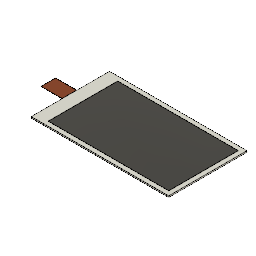
METEOSTANICE VNITRNI SESTAVA v6 (Autodesk Fusion 360 archive; units mm, degrees)
design "E-ink displej"
Autodesk Fusion 360 part; units mm, degrees
(part 1 of 2)
sketch "Sketch1" plane through (0, 0, 0) normal (0, 0, 1) x (1, 0, 0)
  line L0 (0, 0) -> (92.99, 0)
  line L1 (92.99, 0) -> (92.99, 53)
  line L2 (92.99, 53) -> (0, 53)
  line L3 (0, 53) -> (0, 0)
  dimension "d1" = 92.99
  dimension "d2" = 53
  constraint horizontal L0
  constraint vertical L1
  constraint horizontal L2
  constraint vertical L3
  constraint coincident L0.start L3.end
  measures "d1" distance of L0.start L0.end
  measures "d2" distance of L0.start L2.end
extrude "Extrude1" add sketch "Sketch1" along normal blind 1 makes body 1
sketch "Sketch2" plane through (0, 0, 1) normal (0, 0, 1) x (-1, 0, 0)
  line L0 (0, -53) -> (0, 0)
  line L1 (0, 0) -> (-92.99, 0)
  line L2 (-92.99, 0) -> (-92.99, -53)
  line L3 (-92.99, -53) -> (0, -53)
  line L4 (-8.5, -3) -> (-90.04, -3)
  line L5 (-90.04, -3) -> (-90.04, -50.04)
  line L6 (-90.04, -50.04) -> (-8.5, -50.04)
  line L7 (-8.5, -50.04) -> (-8.5, -3)
  dimension "d5" = 81.54
  dimension "d6" = 47.04
  dimension "d7" = 8.5
  dimension "d8" = 3
  constraint horizontal L4
  constraint vertical L5
  constraint horizontal L6
  constraint vertical L7
  measures "d5" distance of L4.start L4.end
  measures "d6" distance of L4.start L6.end
  measures "d7" horizontal distance of L0.end L4.start
  measures "d8" vertical distance of L0.end L4.start
extrude "Extrude2" add sketch "Sketch2" along normal blind 0.001 separate body contours L4 L5 L6 L7 makes body 2
sketch "Sketch3" plane through (0, 0, 0) normal (-1, 0, 0) x (0, -1, 0)
  line L0 (-53, 0) -> (0, 0)
  line L1 (0, 0) -> (0, 1)
  line L2 (0, 1) -> (-53, 1)
  line L3 (-53, 1) -> (-53, 0)
  line L4 (-26.5, 1) -> (-26.5, 0)
  line L5 (-26.5, 0.3186) -> (-21.5, 0.3186)
  line L6 (-21.5, 0.3186) -> (-31.5, 0.3186)
  line L7 (-31.5, 0.3186) -> (-31.5, 0.4186)
  line L8 (-31.5, 0.4186) -> (-21.5, 0.4186)
  line L9 (-21.5, 0.4186) -> (-21.5, 0.3186)
  dimension "d11" = 5
  dimension "d12" = 10
  dimension "d13" = 0.1
  constraint midpoint L2 L4.start
  constraint midpoint L0 L4.end
  constraint coincident L4 L5.start
  constraint perpendicular L4 L5
  constraint horizontal L6
  constraint vertical L7
  constraint horizontal L8
  constraint vertical L9
  measures "d11" distance of L5.start L5.end
  measures "d12" distance of L5.end L6.end
  measures "d13" distance of L5.end L8.end
extrude "Extrude3" add sketch "Sketch3" along normal blind 15 separate body contours L4 L6 L7 L8 | L4 L5 L6 L8 L9 makes body 3

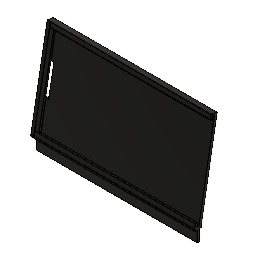
design "meteostanice_vnitrni-uchytDisplej"
Autodesk Fusion 360 part; units mm, degrees
sketch "Sketch1" plane through (0, 0, 0) normal (1, 0, 0) x (0, 1, 0)
  line L0 (0, 0) -> (1.5, 0)
  line L1 (0, 0) -> (0, 6.8)
  line L2 (1.5, 0) -> (1.5, 6.8)
  line L3 (0, 6.8) -> (-1.5, 6.8)
  line L4 (-1.5, 6.8) -> (-1.5, 7.8)
  line L5 (1.5, 6.8) -> (2.5, 6.8)
  line L6 (2.5, 6.8) -> (2.5, 7.8)
  line L7 (2.5, 7.8) -> (-1.5, 7.8)
  line L8 (-1.5, 7.8) -> (-1.0311, 10.459)
  line L9 (-1.0311, 10.459) -> (-0.0463, 10.2853)
  line L10 (2.5, 7.8) -> (11.9465, 61.3735)
  line L11 (2.5, 7.8) -> (56, 7.8) construction
  line L12 (2.5, 7.8) -> (1.0228, 8.0605)
  line L13 (2.5, 7.8) -> (3.5, 7.8) construction
  line L14 (1.0228, 8.0605) -> (10.4692, 61.634)
  line L15 (1.0228, 8.0605) -> (55.0152, 8.0605) construction
  line L16 (11.9465, 61.3735) -> (10.4692, 61.634)
  line L17 (1.0228, 8.0605) -> (-0.159, 8.2689)
  line L18 (-0.159, 8.2689) -> (0.1893, 10.2438)
  line L19 (0.1893, 10.2438) -> (-0.0463, 10.2853)
  line L20 (10.4692, 61.634) -> (9.2875, 61.8424)
  line L21 (9.2875, 61.8424) -> (8.8186, 59.1834)
  line L22 (10.4692, 61.634) -> (10.2956, 60.6492)
  line L23 (10.2956, 60.6492) -> (9.1138, 60.8576)
  line L24 (8.8186, 59.1834) -> (7.8338, 59.3571)
  line L25 (9.2875, 61.8424) -> (8.3027, 62.016)
  line L26 (8.3027, 62.016) -> (7.8338, 59.3571)
  dimension "d1" = 1.5
  dimension "d2" = 6.8
  dimension "d3" = 6.8
  dimension "d4" = 1.5
  dimension "d5" = 1
  dimension "d6" = 1
  dimension "d7" = 1
  dimension "d8" = 2.7
  dimension "d9" = 80
  dimension "d10" = 1
  dimension "d11" = 80
  dimension "d12" = 54.4
  dimension "d13" = 170
  dimension "d14" = 1.5
  dimension "d15" = 80
  dimension "d16" = 54.4
  dimension "d17" = 1.2
  dimension "d18" = 1.2
  dimension "d19" = 2.7
  dimension "d20" = 1
  dimension "d21" = 1
  dimension "d22" = 1
  constraint coincident L0.start L1.start
  constraint horizontal L0
  constraint perpendicular L0 L1
  constraint perpendicular L0 L2
  constraint perpendicular L1 L3
  constraint perpendicular L3 L4
  constraint perpendicular L2 L5
  constraint perpendicular L5 L6
  constraint perpendicular L8 L9
  constraint horizontal L11
  constraint horizontal L13
  constraint horizontal L15
  constraint perpendicular L14 L17
  constraint perpendicular L17 L18
  constraint perpendicular L18 L19
  constraint perpendicular L14 L20
  constraint perpendicular L20 L21
  constraint perpendicular L16 L22
  constraint coincident L21 L23.end
  constraint perpendicular L21 L23
  constraint perpendicular L21 L24
  constraint perpendicular L21 L25
  measures "d1" distance of L0.start L0.end
  measures "d2" distance of L0.start L1.end
  measures "d3" distance of L0.end L2.end
  measures "d4" distance of L1.end L3.end
  measures "d5" distance of L3.end L4.end
  measures "d6" distance of L2.end L5.end
  measures "d7" distance of L5.end L6.end
  measures "d8" distance of L4.end L8.end
  measures "d9" angle of L7 L8
  measures "d10" distance of L8.end L9.end
  measures "d11" angle of L10 L11
  measures "d12" distance of L6.end L10.end
  measures "d13" angle of L12 L13
  measures "d14" distance of L6.end L12.end
  measures "d15" angle of L14 L15
  measures "d16" distance of L12.end L14.end
  measures "d17" distance of L12.end L17.end
  measures "d18" distance of L14.end L20.end
  measures "d19" distance of L20.end L21.end
  measures "d20" distance of L14.end L22.end
  measures "d21" distance of L21.end L24.end
  measures "d22" distance of L20.end L25.end
extrude "Extrude1" add sketch "Sketch1" along normal blind 95.5
sketch "Sketch2" plane through (0, 0, 0) normal (-1, 0, 0) x (0, -1, 0)
  line L0 (-1.5, 0) -> (0, 0)
  line L1 (0, 0) -> (0, 6.8)
  line L2 (0, 6.8) -> (1.5, 6.8)
  line L3 (1.5, 6.8) -> (1.5, 7.8)
  line L4 (1.5, 7.8) -> (1.0311, 10.459)
  line L5 (1.0311, 10.459) -> (-0.1893, 10.2438)
  line L6 (-0.1893, 10.2438) -> (0.159, 8.2689)
  line L7 (0.159, 8.2689) -> (-1.0228, 8.0605)
  line L8 (-1.0228, 8.0605) -> (-10.2956, 60.6492)
  line L9 (-10.2956, 60.6492) -> (-9.1138, 60.8576)
  line L10 (-9.1138, 60.8576) -> (-8.8186, 59.1834)
  line L11 (-8.8186, 59.1834) -> (-7.8338, 59.3571)
  line L12 (-7.8338, 59.3571) -> (-8.3027, 62.016)
  line L13 (-8.3027, 62.016) -> (-11.9465, 61.3735)
  line L14 (-11.9465, 61.3735) -> (-2.5, 7.8)
  line L15 (-2.5, 7.8) -> (-2.5, 6.8)
  line L16 (-2.5, 6.8) -> (-1.5, 6.8)
  line L17 (-1.5, 6.8) -> (-1.5, 0)
  line L18 (1.5, 6.8) -> (-2.5, 6.8)
  line L19 (-2.5, 7.8) -> (-11.9465, 61.3735)
  line L20 (-11.9465, 61.3735) -> (-8.3027, 62.016)
  line L21 (-8.3027, 62.016) -> (1.5, 7.8)
  line L22 (1.5, 7.8) -> (1.5, 6.8)
  constraint coincident L2.end L3.start
  constraint coincident L15.end L16.start
  constraint coincident L14.end L15.start
  constraint coincident L13.end L14.start
  constraint coincident L12.end L13.start
  constraint coincident L3.end L4.start
extrude "Extrude2" add sketch "Sketch2" along normal blind 2 contours L2 L3 L5 L6 L7 L8 L9 L10 L11 L12 L13 L14 L15 L16 L18 L19 L20 L21 L22 | L5 L6 L7 L8 L9 L10 L11 L12 L21
sketch "Sketch3" plane through (0, -0.3865, 0.0681) normal (0, -0.984808, 0.173648) x (1, 0, 0)
  line L0 (0, 61.5156) -> (0, 8.1156)
  line L1 (0, 8.1156) -> (95.5, 8.1156)
  line L2 (95.5, 8.1156) -> (95.5, 61.5156)
  line L3 (95.5, 61.5156) -> (0, 61.5156)
  line L4 (0, 61.5156) -> (0, 8.1156)
  line L5 (0, 34.8156) -> (18, 34.8156)
  line L6 (0, 34.8156) -> (3, 34.8156)
  line L7 (3, 34.8156) -> (3, 25.8156)
  line L8 (3, 25.8156) -> (0, 25.8156)
  line L9 (0, 25.8156) -> (0, 43.8156)
  line L10 (0, 43.8156) -> (3, 43.8156)
  line L11 (3, 43.8156) -> (3, 25.8156)
  dimension "d27" = 9
  dimension "d28" = 3
  dimension "d29" = 18
  constraint coincident L0.start L3.end
  constraint coincident L0.end L1.start
  constraint midpoint L0 L5.start
  constraint perpendicular L0 L5
  constraint coincident L5 L6.end
  constraint perpendicular L5 L7
  constraint horizontal L8
  constraint vertical L9
  constraint horizontal L10
  constraint vertical L11
  measures "d27" distance of L6.end L7.end
  measures "d28" distance of L7.end L8.end
  measures "d29" distance of L7.end L10.end
extrude "Extrude3" cut sketch "Sketch3" against normal blind 4 contours L0 L4 L5 L6 L9 L10 L11 | L0 L4 L5 L6 L7 L8 L9 L11
sketch "Sketch4" plane through (0, 0, 0) normal (1, 0, 0) x (0, 1, 0)
  line L0 (7.8338, 59.3571) -> (8.3027, 62.016)
  line L1 (8.3027, 62.016) -> (-1.0196, 10.4569)
  line L2 (-1.0196, 10.4569) -> (0.1893, 10.2438)
  line L3 (0.1893, 10.2438) -> (-0.159, 8.2689)
  line L4 (-0.159, 8.2689) -> (1.0228, 8.0605)
  line L5 (1.0228, 8.0605) -> (4.0964, 25.4916)
  line L6 (4.0964, 25.4916) -> (5.5736, 25.2311)
  line L7 (5.5736, 25.2311) -> (8.6992, 42.9576)
  line L8 (8.6992, 42.9576) -> (7.222, 43.2181)
  line L9 (7.222, 43.2181) -> (10.2956, 60.6492)
  line L10 (10.2956, 60.6492) -> (9.1138, 60.8576)
  line L11 (9.1138, 60.8576) -> (8.8186, 59.1834)
  line L12 (8.8186, 59.1834) -> (7.8338, 59.3571)
  line L13 (-1.0196, 10.4569) -> (0.1893, 10.2438)
  line L14 (0.1893, 10.2438) -> (8.8186, 59.1834)
  line L15 (8.8186, 59.1834) -> (7.8338, 59.3571)
  line L16 (7.8338, 59.3571) -> (-1.0196, 10.4569)
  constraint coincident L1.end L2.start
  constraint coincident L2.end L3.start
  constraint coincident L11.end L12.start
  constraint coincident L0.start L12.end
extrude "Extrude4" add sketch "Sketch4" along normal blind 2.5 contours L2 L12 L13 L14 L15 L16
sketch "Sketch5" plane through (0, 0, 0) normal (1, 0, 0) x (0, 1, 0)
  line L0 (9.1138, 60.8576) -> (-0.159, 8.2689)
  line L1 (-0.159, 8.2689) -> (1.0228, 8.0605)
  line L2 (1.0228, 8.0605) -> (4.0964, 25.4916)
  line L3 (4.0964, 25.4916) -> (5.5736, 25.2311)
  line L4 (5.5736, 25.2311) -> (8.6992, 42.9576)
  line L5 (8.6992, 42.9576) -> (7.222, 43.2181)
  line L6 (7.222, 43.2181) -> (10.2956, 60.6492)
  line L7 (10.2956, 60.6492) -> (9.1138, 60.8576)
  line L8 (8.6992, 42.9576) -> (5.5736, 25.2311)
  line L9 (7.1364, 34.0944) -> (12.0604, 33.2261)
  line L10 (7.1364, 34.0944) -> (9.0899, 45.1735)
  line L11 (7.1364, 34.0944) -> (18.3864, 34.0944) construction
  line L12 (9.0899, 45.1735) -> (9.3504, 46.6507)
  line L13 (9.3504, 46.6507) -> (16.7365, 45.3483)
  line L14 (16.7365, 45.3483) -> (15.6946, 39.4395)
  line L15 (15.6946, 39.4395) -> (14.2174, 39.6999)
  line L16 (14.2174, 39.6999) -> (14.9988, 44.1316)
  line L17 (14.9988, 44.1316) -> (9.0899, 45.1735)
  line L18 (5.1829, 23.0153) -> (4.9224, 21.5381)
  line L19 (11.0917, 21.9734) -> (5.1829, 23.0153)
  line L20 (4.9224, 21.5381) -> (12.3085, 20.2357)
  line L21 (12.3085, 20.2357) -> (13.3503, 26.1446)
  line L22 (11.8731, 26.405) -> (11.0917, 21.9734)
  line L23 (13.3503, 26.1446) -> (11.8731, 26.405)
  dimension "d34" = 5
  dimension "d35" = 80
  dimension "d36" = 11.25
  dimension "d37" = 1.5
  dimension "d38" = 7.5
  dimension "d39" = 6
  dimension "d40" = 1.5
  dimension "d41" = 4.5
  constraint coincident L4.end L5.start
  constraint coincident L3.end L4.start
  constraint midpoint L4 L9.start
  constraint perpendicular L4 L9
  constraint horizontal L11
  constraint parallel L10 L12
  constraint perpendicular L12 L13
  constraint perpendicular L13 L14
  constraint perpendicular L14 L15
  constraint perpendicular L15 L16
  constraint symmetric L9 L10.end L18.start
  constraint symmetric L9 L12.end L18.end
  constraint symmetric L9 L13.end L20.end
  constraint symmetric L9 L14.end L21.end
  constraint symmetric L9 L15.end L22.start
  constraint symmetric L9 L16.end L19.start
  measures "d34" distance of L9.start L9.end
  measures "d35" angle of L10 L11
  measures "d36" distance of L9.start L10.end
  measures "d37" distance of L10.end L12.end
  measures "d38" distance of L12.end L13.end
  measures "d39" distance of L13.end L14.end
  measures "d40" distance of L14.end L15.end
  measures "d41" distance of L15.end L16.end
extrude "Extrude5" add sketch "Sketch5" along normal blind 65 and the other way blind 2 contours L12 L13 L14 L15 L16 L17 | L18 L19 L20 L21 L22 L23
sketch "Sketch6" plane through (0, 1.0907, -0.1923) normal (0, 0.984808, -0.173648) x (-1, 0, 0)
  line L0 (0, 43.8156) -> (0, 25.8156)
  line L1 (0, 25.8156) -> (-3, 25.8156)
  line L2 (-3, 25.8156) -> (-3, 43.8156)
  line L3 (-3, 43.8156) -> (0, 43.8156)
  line L4 (2, 22.0656) -> (-65, 22.0656)
  line L5 (-65, 22.0656) -> (-65, 23.5656)
  line L6 (-65, 23.5656) -> (2, 23.5656)
  line L7 (2, 23.5656) -> (2, 46.0656)
  line L8 (2, 46.0656) -> (-65, 46.0656)
  line L9 (-65, 46.0656) -> (-65, 47.5656)
  line L10 (-65, 47.5656) -> (2, 47.5656)
  line L11 (2, 47.5656) -> (2, 62.5156)
  line L12 (2, 62.5156) -> (-95.5, 62.5156)
  line L13 (-95.5, 62.5156) -> (-95.5, 8.1156)
  line L14 (-95.5, 8.1156) -> (2, 8.1156)
  line L15 (2, 8.1156) -> (2, 22.0656)
  line L16 (2, 46.0656) -> (1, 46.0656)
  line L17 (1, 46.0656) -> (1, 23.5656)
  line L18 (1, 23.5656) -> (2, 23.5656)
  line L19 (2, 23.5656) -> (2, 46.0656)
  dimension "d46" = 1
  dimension "d47" = 22.5
  constraint horizontal L16
  constraint vertical L17
  constraint horizontal L18
  constraint vertical L19
  constraint coincident L7.end L8.start
  measures "d46" distance of L7.end L16.end
  measures "d47" distance of L7.end L6.end
extrude "Extrude6" add sketch "Sketch6" along normal blind 6 contours L6 L7 L8 L16 L17 L18 L19
sketch "Sketch7" plane through (-2, 0, 0) normal (-1, 0, 0) x (0, -1, 0)
  line L0 (-2.5, 7.8) -> (-2.5, 6.8)
  line L1 (-2.5, 6.8) -> (1.5, 6.8)
  line L2 (1.5, 6.8) -> (1.5, 7.8)
  line L3 (1.5, 7.8) -> (-8.3027, 62.016)
  line L4 (-8.3027, 62.016) -> (-11.9465, 61.3735)
  line L5 (-11.9465, 61.3735) -> (-9.3504, 46.6507)
  line L6 (-9.3504, 46.6507) -> (-16.7365, 45.3483)
  line L7 (-16.7365, 45.3483) -> (-15.6946, 39.4395)
  line L8 (-15.6946, 39.4395) -> (-14.2174, 39.6999)
  line L9 (-14.2174, 39.6999) -> (-11.8731, 26.405)
  line L10 (-11.8731, 26.405) -> (-13.3503, 26.1446)
  line L11 (-13.3503, 26.1446) -> (-12.3085, 20.2357)
  line L12 (-12.3085, 20.2357) -> (-4.9224, 21.5381)
  line L13 (-4.9224, 21.5381) -> (-2.5, 7.8)
  line L14 (-9.3504, 46.6507) -> (-4.9224, 21.5381)
  line L15 (-9.3504, 46.6507) -> (-18.5206, 45.0337)
  line L16 (-18.5206, 45.0337) -> (-12.3085, 20.2357)
  line L17 (-4.9224, 21.5381) -> (-12.3085, 20.2357)
  constraint coincident L5.end L6.start
  constraint coincident L12.end L13.start
  constraint perpendicular L7 L15
  constraint coincident L11.end L12.start
extrude "Extrude7" cut sketch "Sketch7" against normal blind 2 contours L6 L7 L8 L9 L10 L11 L12 L14 L15 L17 | L7 L8 L9 L10 L11 L15 L16
equation "d27 = ( 18 / 2 ) * 1 mm"
equation "d36 = ( 22.5 / 2 ) * 1 mm"
equation "d41 = 6 mm - 1.5 mm"

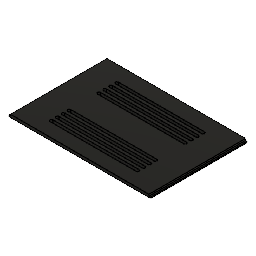
design "meteostanice_vnitrni-viko"
Autodesk Fusion 360 part; units mm, degrees
sketch "Sketch4" plane through (0, 0, 0) normal (0, 0, 1) x (1, 0, 0)
  line L0 (0, 0) -> (95.5, 0)
  line L1 (95.5, 0) -> (95.5, 65.054)
  line L2 (95.5, 65.054) -> (0, 65.054)
  line L3 (0, 65.054) -> (0, 0)
  dimension "d32" = 95.5
  dimension "d33" = 65.054
  constraint horizontal L0
  constraint vertical L1
  constraint horizontal L2
  constraint vertical L3
  constraint coincident L0.start L3.end
  measures "d32" distance of L0.start L0.end
  measures "d33" distance of L0.start L2.end
extrude "Extrude4" add sketch "Sketch4" along normal blind 0.9
sketch "Sketch5" plane through (0, 0, 0.9) normal (0, 0, 1) x (-1, 0, 0)
  line L0 (0, -65.054) -> (0, 0)
  line L1 (0, 0) -> (-95.5, 0)
  line L2 (-95.5, 0) -> (-95.5, -65.054)
  line L3 (-95.5, -65.054) -> (0, -65.054)
  line L4 (0, 0) -> (-1.1, 0)
  line L5 (-95.5, -65.054) -> (-94.4, -65.054)
  line L6 (-1.1, 0) -> (-94.4, 0)
  line L7 (-94.4, 0) -> (-94.4, -65.054)
  line L8 (-94.4, -65.054) -> (-1.1, -65.054)
  line L9 (-1.1, -65.054) -> (-1.1, 0)
  dimension "d36" = 1.1
  dimension "d37" = 1.1
  constraint coincident L0.end L1.start
  constraint horizontal L4
  constraint coincident L2.end L3.start
  constraint perpendicular L2 L5
  constraint horizontal L6
  constraint vertical L7
  constraint horizontal L8
  constraint vertical L9
  measures "d36" distance of L0.end L4.end
  measures "d37" distance of L2.end L5.end
extrude "Extrude5" add sketch "Sketch5" along normal blind 1.1 contours L1 L3 L6 L7 L8 L9
sketch "Sketch6" plane through (0, 0, 2) normal (0, 0, 1) x (-1, 0, 0)
  line L0 (-1.1, -65.054) -> (-1.1, 0)
  line L1 (-1.1, 0) -> (-94.4, 0)
  line L2 (-94.4, 0) -> (-94.4, -65.054)
  line L3 (-94.4, -65.054) -> (-1.1, -65.054)
  line L4 (-47.75, -65.054) -> (-47.75, -55.054)
  line L5 (-47.75, -55.054) -> (-77.75, -55.054)
  line L6 (-76.75, -55.054) -> (-18.75, -55.054)
  line L7 (-18.75, -53.054) -> (-76.75, -53.054)
  arc A0 (-18.75, -55.054) -> (-17.75, -54.054) centre (-18.75, -54.054) ccw
  arc A1 (-17.75, -54.054) -> (-18.75, -53.054) centre (-18.75, -54.054) ccw
  arc A2 (-77.75, -54.054) -> (-76.75, -55.054) centre (-76.75, -54.054) ccw
  arc A3 (-76.75, -53.054) -> (-77.75, -54.054) centre (-76.75, -54.054) ccw
  line L8 (-18.75, -49.054) -> (-76.75, -49.054)
  arc A4 (-76.75, -49.054) -> (-77.75, -50.054) centre (-76.75, -50.054) ccw
  line L9 (-47.75, -51.054) -> (-77.75, -51.054)
  arc A5 (-77.75, -50.054) -> (-76.75, -51.054) centre (-76.75, -50.054) ccw
  arc A6 (-18.75, -51.054) -> (-17.75, -50.054) centre (-18.75, -50.054) ccw
  arc A7 (-17.75, -50.054) -> (-18.75, -49.054) centre (-18.75, -50.054) ccw
  line L10 (-76.75, -51.054) -> (-18.75, -51.054)
  line L11 (-76.75, -43.054) -> (-18.75, -43.054)
  arc A8 (-17.75, -46.054) -> (-18.75, -45.054) centre (-18.75, -46.054) ccw
  arc A9 (-18.75, -43.054) -> (-17.75, -42.054) centre (-18.75, -42.054) ccw
  line L12 (-47.75, -47.054) -> (-77.75, -47.054)
  arc A10 (-77.75, -46.054) -> (-76.75, -47.054) centre (-76.75, -46.054) ccw
  arc A11 (-18.75, -47.054) -> (-17.75, -46.054) centre (-18.75, -46.054) ccw
  line L13 (-47.75, -43.054) -> (-77.75, -43.054)
  arc A12 (-76.75, -45.054) -> (-77.75, -46.054) centre (-76.75, -46.054) ccw
  arc A13 (-77.75, -42.054) -> (-76.75, -43.054) centre (-76.75, -42.054) ccw
  line L14 (-18.75, -45.054) -> (-76.75, -45.054)
  line L15 (-76.75, -47.054) -> (-18.75, -47.054)
  line L16 (-18.75, -41.054) -> (-76.75, -41.054)
  arc A14 (-17.75, -42.054) -> (-18.75, -41.054) centre (-18.75, -42.054) ccw
  arc A15 (-76.75, -41.054) -> (-77.75, -42.054) centre (-76.75, -42.054) ccw
  arc A16 (-76.75, -13.054) -> (-77.75, -14.054) centre (-76.75, -14.054) ccw
  arc A17 (-17.75, -14.054) -> (-18.75, -13.054) centre (-18.75, -14.054) ccw
  line L17 (-76.75, -11.054) -> (-18.75, -11.054)
  arc A18 (-18.75, -11.054) -> (-17.75, -10.054) centre (-18.75, -10.054) ccw
  line L18 (-47.75, -23.054) -> (-77.75, -23.054)
  arc A19 (-17.75, -10.054) -> (-18.75, -9.054) centre (-18.75, -10.054) ccw
  arc A20 (-18.75, -15.054) -> (-17.75, -14.054) centre (-18.75, -14.054) ccw
  arc A21 (-77.75, -22.054) -> (-76.75, -23.054) centre (-76.75, -22.054) ccw
  line L19 (-47.75, -11.054) -> (-77.75, -11.054)
  arc A22 (-77.75, -18.054) -> (-76.75, -19.054) centre (-76.75, -18.054) ccw
  arc A23 (-17.75, -18.054) -> (-18.75, -17.054) centre (-18.75, -18.054) ccw
  arc A24 (-18.75, -23.054) -> (-17.75, -22.054) centre (-18.75, -22.054) ccw
  arc A25 (-76.75, -21.054) -> (-77.75, -22.054) centre (-76.75, -22.054) ccw
  arc A26 (-77.75, -10.054) -> (-76.75, -11.054) centre (-76.75, -10.054) ccw
  line L20 (-76.75, -15.054) -> (-18.75, -15.054)
  line L21 (-47.75, -19.054) -> (-77.75, -19.054)
  line L22 (-18.75, -9.054) -> (-76.75, -9.054)
  line L23 (-76.75, -23.054) -> (-18.75, -23.054)
  line L24 (-18.75, -13.054) -> (-76.75, -13.054)
  line L25 (-18.75, -17.054) -> (-76.75, -17.054)
  arc A27 (-77.75, -14.054) -> (-76.75, -15.054) centre (-76.75, -14.054) ccw
  arc A28 (-76.75, -9.054) -> (-77.75, -10.054) centre (-76.75, -10.054) ccw
  arc A29 (-17.75, -22.054) -> (-18.75, -21.054) centre (-18.75, -22.054) ccw
  arc A30 (-76.75, -17.054) -> (-77.75, -18.054) centre (-76.75, -18.054) ccw
  line L26 (-76.75, -19.054) -> (-18.75, -19.054)
  line L27 (-47.75, -15.054) -> (-77.75, -15.054)
  line L28 (-18.75, -21.054) -> (-76.75, -21.054)
  arc A31 (-18.75, -19.054) -> (-17.75, -18.054) centre (-18.75, -18.054) ccw
  point P0 (-17.75, -55.054)
  point P1 (-77.75, -53.054)
  point P2 (-17.75, -51.054)
  point P3 (-77.75, -49.054)
  point P4 (-17.75, -47.054)
  point P5 (-77.75, -45.054)
  point P6 (-17.75, -43.054)
  point P7 (-77.75, -41.054)
  point P8 (-17.75, -23.054)
  point P9 (-77.75, -21.054)
  point P10 (-17.75, -19.054)
  point P11 (-77.75, -17.054)
  point P12 (-17.75, -15.054)
  point P13 (-77.75, -13.054)
  point P14 (-17.75, -11.054)
  point P15 (-77.75, -9.054)
  dimension "d40" = 10
  dimension "d41" = 30
  dimension "d42" = 60
  dimension "d43" = 2
  dimension "d44" = 1
  dimension "d45" = 30
  dimension "d46" = 60
  dimension "d47" = 2
  dimension "d48" = 1
  dimension "d49" = 30
  dimension "d50" = 60
  dimension "d51" = 2
  dimension "d52" = 1
  dimension "d53" = 30
  dimension "d54" = 60
  dimension "d55" = 2
  dimension "d56" = 1
  dimension "d57" = 30
  dimension "d58" = 60
  dimension "d59" = 2
  dimension "d60" = 1
  dimension "d61" = 30
  dimension "d62" = 60
  dimension "d63" = 2
  dimension "d64" = 1
  dimension "d65" = 30
  dimension "d66" = 60
  dimension "d67" = 2
  dimension "d68" = 1
  dimension "d69" = 30
  dimension "d70" = 60
  dimension "d71" = 2
  dimension "d72" = 1
  constraint midpoint L3 L4.start
  constraint perpendicular L3 L4
  constraint perpendicular L4 L5
  constraint horizontal L6
  constraint horizontal L7
  constraint coincident P0 L6
  constraint tangent L6 A0
  constraint tangent L7 A1
  constraint equal A0 A1
  constraint coincident A0.end A1.start
  constraint coincident L5.end L6
  constraint tangent L6 A2
  constraint equal A0 A2
  constraint coincident P1 L7
  constraint tangent L7 A3
  constraint equal A0 A3
  constraint coincident A2.start A3.end
  constraint horizontal L10
  constraint horizontal L8
  constraint coincident P2 L10
  constraint tangent A6 L10
  constraint tangent L8 A7
  constraint equal A6 A7
  constraint coincident A6.end A7.start
  constraint coincident L9.end L10
  constraint tangent A5 L10
  constraint equal A5 A6
  constraint coincident P3 L8
  constraint tangent L8 A4
  constraint equal A4 A6
  constraint coincident A4.end A5.start
  constraint horizontal L15
  constraint horizontal L14
  constraint coincident P4 L15
  constraint tangent A11 L15
  constraint tangent A8 L14
  constraint equal A8 A11
  constraint coincident A8.start A11.end
  constraint coincident L12.end L15
  constraint tangent A10 L15
  constraint equal A10 A11
  constraint coincident P5 L14
  constraint tangent A12 L14
  constraint equal A11 A12
  constraint coincident A10.start A12.end
  constraint horizontal L11
  constraint horizontal L16
  constraint coincident P6 L11
  constraint tangent L11 A9
  constraint tangent L16 A14
  constraint equal A9 A14
  constraint coincident A9.end A14.start
  constraint coincident L13.end L11
  constraint tangent L11 A13
  constraint equal A9 A13
  constraint coincident P7 L16
  constraint tangent L16 A15
  constraint equal A9 A15
  constraint coincident A13.start A15.end
  constraint horizontal L23
  constraint horizontal L28
  constraint coincident P8 L23
  constraint tangent A24 L23
  constraint tangent A29 L28
  constraint equal A24 A29
  constraint coincident A24.end A29.start
  constraint coincident L18.end L23
  constraint tangent A21 L23
  constraint equal A21 A24
  constraint coincident P9 L28
  constraint tangent A25 L28
  constraint equal A24 A25
  constraint coincident A21.start A25.end
  constraint horizontal L26
  constraint horizontal L25
  constraint coincident P10 L26
  constraint tangent L26 A31
  constraint tangent A23 L25
  constraint equal A23 A31
  constraint coincident A23.start A31.end
  constraint coincident L21.end L26
  constraint tangent A22 L26
  constraint equal A22 A31
  constraint coincident P11 L25
  constraint tangent L25 A30
  constraint equal A30 A31
  constraint coincident A22.start A30.end
  constraint horizontal L20
  constraint horizontal L24
  constraint coincident P12 L20
  constraint tangent A20 L20
  constraint tangent A17 L24
  constraint equal A17 A20
  constraint coincident A17.start A20.end
  constraint coincident L27.end L20
  constraint tangent L20 A27
  constraint equal A20 A27
  constraint coincident P13 L24
  constraint tangent A16 L24
  constraint equal A16 A20
  constraint coincident A16.end A27.start
  constraint horizontal L17
  constraint horizontal L22
  constraint coincident P14 L17
  constraint tangent L17 A18
  constraint tangent A19 L22
  constraint equal A18 A19
  constraint coincident A18.end A19.start
  constraint coincident L19.end L17
  constraint tangent L17 A26
  constraint equal A18 A26
  constraint coincident P15 L22
  constraint tangent L22 A28
  constraint equal A18 A28
  constraint coincident A26.start A28.end
  measures "d40" distance of L4.start L4.end
  measures "d41" distance of L4.end L5.end
  measures "d42" distance of L5.end P0
  measures "d43" distance of L5.end P1
  measures "d44" radius of A0
  measures "d45" distance of L9.end L9.start
  measures "d46" distance of L9.end P2
  measures "d47" distance of L9.end P3
  measures "d48" radius of A6
  measures "d49" distance of L12.end L12.start
  measures "d50" distance of L12.end P4
  measures "d51" distance of L12.end P5
  measures "d52" radius of A11
  measures "d53" distance of L13.end L13.start
  measures "d54" distance of L13.end P6
  measures "d55" distance of L13.end P7
  measures "d56" radius of A9
  measures "d57" distance of L18.end L18.start
  measures "d58" distance of L18.end P8
  measures "d59" distance of L18.end P9
  measures "d60" radius of A24
  measures "d61" distance of L21.end L21.start
  measures "d62" distance of L21.end P10
  measures "d63" distance of L21.end P11
  measures "d64" radius of A31
  measures "d65" distance of L27.end L27.start
  measures "d66" distance of L27.end P12
  measures "d67" distance of L27.end P13
  measures "d68" radius of A20
  measures "d69" distance of L19.start L19.end
  measures "d70" distance of L19.end P14
  measures "d71" distance of L19.end P15
  measures "d72" radius of A18
extrude "Extrude6" cut sketch "Sketch6" against normal blind 5 contours L5 L6 L7 A0 A1 A2 A3 | L8 A4 L9 A5 A6 A7 L10 | L11 A9 L13 A13 L16 A14 A15 | A8 L12 A10 A11 A12 L14 L15 | A16 A17 A20 L20 L24 A27 L27 | L17 A18 A19 L19 A26 L22 A28 | L18 A21 A24 A25 L23 A29 L28 | A22 A23 L21 L25 A30 L26 A31

design "meteostanice_vnitrni-krabicka"
Autodesk Fusion 360 part; units mm, degrees
sketch "Sketch1" plane through (0, 0, 0) normal (0, 0, 1) x (1, 0, 0)
  line L0 (0, 0) -> (57, 0)
  line L1 (57, 0) -> (57, 70)
  line L2 (57, 70) -> (0, 70)
  line L3 (0, 70) -> (0, 0)
  circle A0 centre (53.25, 66.25) radius 1.6
  circle A1 centre (53.25, 3.75) radius 1.6
  circle A2 centre (7.25, 32.75) radius 1.6
  line L4 (57, 70) -> (57.5, 70)
  line L5 (57.5, 70) -> (57.5, 70.5)
  line L6 (57.5, 70.5) -> (57, 70.5)
  line L7 (57, 70.5) -> (57, 70)
  line L8 (0, 0) -> (-0.5, 0)
  line L9 (-0.5, 0) -> (-0.5, -0.5)
  line L10 (-0.5, -0.5) -> (0, -0.5)
  line L11 (0, -0.5) -> (0, 0)
  line L12 (-0.5, -0.5) -> (57.5, -0.5)
  line L13 (57.5, -0.5) -> (57.5, 70.5)
  line L14 (57.5, 70.5) -> (-0.5, 70.5)
  line L15 (-0.5, 70.5) -> (-0.5, -0.5)
  line L16 (-0.5, -0.5) -> (93, -0.5)
  line L17 (93, -0.5) -> (93, 71)
  line L18 (93, 71) -> (-0.5, 71)
  line L19 (-0.5, 71) -> (-0.5, -0.5)
  line L20 (-0.5, -0.5) -> (-2.5, -0.5)
  line L21 (-2.5, -0.5) -> (-2.5, -2.5)
  line L22 (-2.5, -2.5) -> (-0.5, -2.5)
  line L23 (-0.5, -2.5) -> (-0.5, -0.5)
  line L24 (93, 71) -> (95, 71)
  line L25 (95, 71) -> (95, 73)
  line L26 (95, 73) -> (93, 73)
  line L27 (93, 73) -> (93, 71)
  line L28 (-2.5, -2.5) -> (95, -2.5)
  line L29 (95, -2.5) -> (95, 73)
  line L30 (95, 73) -> (-2.5, 73)
  line L31 (-2.5, 73) -> (-2.5, -2.5)
  dimension "d11" = 57
  dimension "d12" = 70
  dimension "d13" = 3.2
  dimension "d14" = 3.75
  dimension "d15" = 3.75
  dimension "d16" = 3.2
  dimension "d17" = 62.5
  dimension "d18" = 3.75
  dimension "d19" = 3.2
  dimension "d20" = 46
  dimension "d21" = 29
  dimension "d22" = 0.5
  dimension "d23" = 0.5
  dimension "d24" = 0.5
  dimension "d25" = 0.5
  dimension "d26" = 2
  dimension "d27" = 2
  dimension "d28" = 2
  dimension "d29" = 2
  constraint horizontal L0
  constraint vertical L1
  constraint horizontal L2
  constraint vertical L3
  constraint coincident L0.start L3.end
  constraint horizontal L4
  constraint vertical L5
  constraint horizontal L6
  constraint vertical L7
  constraint horizontal L8
  constraint vertical L9
  constraint horizontal L10
  constraint vertical L11
  constraint horizontal L12
  constraint vertical L13
  constraint horizontal L14
  constraint vertical L15
  constraint horizontal L16
  constraint vertical L17
  constraint horizontal L18
  constraint vertical L19
  constraint horizontal L20
  constraint vertical L21
  constraint horizontal L22
  constraint vertical L23
  constraint horizontal L24
  constraint vertical L25
  constraint horizontal L26
  constraint vertical L27
  constraint horizontal L28
  constraint vertical L29
  constraint horizontal L30
  constraint vertical L31
  measures "d11" distance of L0.start L0.end
  measures "d12" distance of L0.start L2.end
  measures "d13" diameter of A0
  measures "d14" vertical distance of L1.end A0.centre
  measures "d15" horizontal distance of L1.end A0.centre
  measures "d16" diameter of A1
  measures "d17" distance of A0.centre A1.centre
  measures "d18" horizontal distance of L0.end A1.centre
  measures "d19" diameter of A2
  measures "d20" horizontal distance of A1.centre A2.centre
  measures "d21" vertical distance of A1.centre A2.centre
  measures "d22" distance of L1.end L4.end
  measures "d23" distance of L1.end L6.end
  measures "d24" distance of L0.start L8.end
  measures "d25" distance of L0.start L10.end
  measures "d26" distance of L9.end L20.end
  measures "d27" distance of L9.end L22.end
  measures "d28" distance of L17.end L24.end
  measures "d29" distance of L17.end L26.end
extrude "Extrude1" add sketch "Sketch1" along normal blind 2 contours L0 L1 L2 L3 | L2 L3 L7 L8 L14 L15 L19 | L8 L9 L10 L11 L12 L15 L16 L19 | L0 L1 L4 L11 L12 L13 L16 | L9 L15 L18 L19 L20 L27 L30 L31 | L10 L12 L16 L17 L23 L24 L28 L29 | L4 L5 L6 L7 L13 L14 | L20 L21 L22 L23 L28 L31 | L5 L6 L13 L14 L16 L17 L18 L19 | L24 L25 L26 L27 L29 L30 | A0 | A1 | A2
sketch "Sketch2" plane through (0, 0, 2) normal (0, 0, 1) x (-1, 0, 0)
  line L0 (2.5, -73) -> (2.5, 2.5)
  line L1 (2.5, 2.5) -> (-95, 2.5)
  line L2 (-95, 2.5) -> (-95, -73)
  line L3 (-95, -73) -> (2.5, -73)
  circle A0 centre (-7.25, -32.75) radius 2.5
  circle A1 centre (-7.25, -32.75) radius 0.75
  circle A2 centre (-53.25, -66.25) radius 2.5
  circle A3 centre (-53.25, -66.25) radius 0.75
  circle A4 centre (-53.25, -3.75) radius 2.5
  circle A5 centre (-53.25, -3.75) radius 0.75
  line L4 (2.5, 2.5) -> (0.5, 2.5)
  line L5 (0.5, 2.5) -> (0.5, 0.5)
  line L6 (0.5, 0.5) -> (2.5, 0.5)
  line L7 (2.5, 0.5) -> (2.5, 2.5)
  line L8 (2.5, 2.5) -> (-95, 2.5)
  line L9 (-95, 2.5) -> (-95, -73)
  line L10 (-95, -73) -> (2.5, -73)
  line L11 (2.5, -73) -> (2.5, 2.5)
  line L12 (-95, -73) -> (-93, -73)
  line L13 (-93, -73) -> (-93, -71)
  line L14 (-93, -71) -> (-95, -71)
  line L15 (-95, -71) -> (-95, -73)
  line L16 (0.5, 0.5) -> (-93, 0.5)
  line L17 (-93, 0.5) -> (-93, -71)
  line L18 (-93, -71) -> (0.5, -71)
  line L19 (0.5, -71) -> (0.5, 0.5)
  dimension "d32" = 5
  dimension "d33" = 1.5
  dimension "d34" = 5
  dimension "d35" = 1.5
  dimension "d36" = 5
  dimension "d37" = 1.5
  dimension "d42" = 2
  dimension "d43" = 2
  dimension "d44" = 2
  dimension "d45" = 2
  constraint concentric A0 A1
  constraint concentric A2 A3
  constraint concentric A4 A5
  constraint horizontal L4
  constraint vertical L5
  constraint horizontal L6
  constraint vertical L7
  constraint coincident L0.end L1.start
  constraint horizontal L8
  constraint vertical L9
  constraint horizontal L10
  constraint vertical L11
  constraint coincident L2.end L3.start
  constraint horizontal L12
  constraint vertical L13
  constraint horizontal L14
  constraint vertical L15
  constraint horizontal L16
  constraint vertical L17
  constraint horizontal L18
  constraint vertical L19
  measures "d32" diameter of A0
  measures "d33" diameter of A1
  measures "d34" diameter of A2
  measures "d35" diameter of A3
  measures "d36" diameter of A4
  measures "d37" diameter of A5
  measures "d42" distance of L0.end L4.end
  measures "d43" distance of L0.end L6.end
  measures "d44" distance of L2.end L12.end
  measures "d45" distance of L2.end L14.end
extrude "Extrude2" add sketch "Sketch2" along normal blind 5 contours A0 | A2 | A4
fillet "Fillet1" radius 1.75 tangency weight 0.96853 3 edges at (9.5808, 31.846, 2) (55.5808, 65.346, 2) (55.5808, 2.846, 2)
extrude "Extrude3" add sketch "Sketch2" along normal blind 32 contours L0 L3 L6 L10 L11 L13 L18 L19 | L0 L1 L4 L5 L6 L7 L8 L11 | L2 L3 L9 L10 L12 L13 L14 L15 | L1 L2 L5 L8 L9 L14 L16 L17
sketch "Sketch3" plane through (0, -0.5, 0) normal (0, 1, 0) x (-1, 0, 0)
  line L0 (-93, 2) -> (-53.2508, 2)
  line L1 (-53.2508, 2) -> (0.5, 2)
  line L2 (0.5, 2) -> (0.5, 34)
  line L3 (0.5, 34) -> (-93, 34)
  line L4 (-93, 34) -> (-93, 2)
  line L5 (-53.2508, 2) -> (-53.2508, 27.5)
  line L6 (-53.2508, 27.5) -> (-47.2508, 27.5)
  line L7 (-47.2508, 27.5) -> (-22.7508, 27.5)
  line L8 (-22.7508, 27.5) -> (-22.7508, 23.5)
  line L9 (-22.7508, 23.5) -> (-47.2508, 23.5)
  line L10 (-47.2508, 23.5) -> (-47.2508, 27.5)
  dimension "d48" = 25.5
  dimension "d49" = 6
  dimension "d50" = 24.5
  dimension "d51" = 4
  constraint coincident L0.end L1.start
  constraint perpendicular L1 L5
  constraint perpendicular L5 L6
  constraint horizontal L7
  constraint vertical L8
  constraint horizontal L9
  constraint vertical L10
  measures "d48" distance of L0.end L5.end
  measures "d49" distance of L5.end L6.end
  measures "d50" distance of L6.end L7.end
  measures "d51" distance of L6.end L9.end
extrude "Extrude4" cut sketch "Sketch3" against normal blind 35 contours L7 L8 L9 L10
chamfer "Chamfer1" distance 4 distance2 1.5 4 edges at (47.2508, -2.5, 25.5) (35.0008, -2.5, 27.5) (22.7508, -2.5, 25.5) (35.0008, -2.5, 23.5) measured on face at (79.0836, -2.5, 19.1667) measured on face at (79.0836, -2.5, 19.1667) measured on face at (79.0836, -2.5, 19.1667) measured on face at (79.0836, -2.5, 19.1667)
sketch "Sketch4" plane through (0, 0, 2) normal (0, 0, 1) x (-1, 0, 0)
  spline S0 degree 3 poles (-57.5, -3.75) (-57.5, -4.8214) (-57.0766, -5.8872) (-55.6545, -7.3945) (-54.7032, -7.8673) (-52.6712, -8.0877) (-51.5959, -7.8015) (-49.9532, -6.6081) (-49.3675, -5.7408) (-48.879, -3.7915) (-49.0041, -2.711) (-49.8812, -1.0097) (-50.5464, -0.3517) (-51.9328, 0.3441) (-52.5917, 0.5001) (-53.2508, 0.5) knots -2.658203 -2.658203 -2.658203 -2.658203 -2.338234 -2.338234 -2.039357 -2.039357 -1.727845 -1.727845 -1.432975 -1.432975 -1.127717 -1.127717 -0.861349 -0.861349 -0.664467 -0.664467 -0.664467 -0.664467
  spline S1 degree 3 poles (-53.2508, 0.5) (-53.4583, 0.5) (-53.6659, 0.4847) (-54.6621, 0.3375) (-55.4178, -0.008) (-56.5915, -1.0189) (-57.0263, -1.6611) (-57.4218, -2.8131) (-57.5, -3.2815) (-57.5, -3.75) knots -0.664467 -0.664467 -0.664467 -0.664467 -0.602484 -0.602484 -0.363754 -0.363754 -0.139905 -0.139905 0 0 0 0
  line L0 (-53.2508, 0.5) -> (-93, 0.5)
  line L1 (-93, 0.5) -> (-93, -71)
  line L2 (-93, -71) -> (0.5, -71)
  line L3 (0.5, -71) -> (0.5, 0.5)
  line L4 (0.5, 0.5) -> (-53.2508, 0.5)
  spline S2 degree 3 poles (-11.5, -32.75) (-11.5, -33.8214) (-11.0766, -34.8872) (-9.6545, -36.3945) (-8.7032, -36.8673) (-6.6712, -37.0877) (-5.5959, -36.8015) (-3.9532, -35.6081) (-3.3675, -34.7408) (-2.879, -32.7915) (-3.0041, -31.711) (-3.8812, -30.0097) (-4.5464, -29.3517) (-6.1183, -28.5627) (-7.0138, -28.4189) (-8.6621, -28.6625) (-9.4178, -29.008) (-10.5915, -30.0189) (-11.0263, -30.6611) (-11.4218, -31.8131) (-11.5, -32.2815) (-11.5, -32.75) knots -2.658203 -2.658203 -2.658203 -2.658203 -2.338234 -2.338234 -2.039357 -2.039357 -1.727845 -1.727845 -1.432975 -1.432975 -1.127717 -1.127717 -0.861349 -0.861349 -0.602484 -0.602484 -0.363754 -0.363754 -0.139905 -0.139905 0 0 0 0
  spline S3 degree 3 poles (-57.5, -66.25) (-57.5, -67.3214) (-57.0766, -68.3872) (-55.6545, -69.8945) (-54.7032, -70.3673) (-52.6712, -70.5877) (-51.5959, -70.3015) (-49.9532, -69.1081) (-49.3675, -68.2408) (-48.879, -66.2915) (-49.0041, -65.211) (-49.8812, -63.5097) (-50.5464, -62.8517) (-52.1183, -62.0627) (-53.0138, -61.9189) (-54.6621, -62.1625) (-55.4178, -62.508) (-56.5915, -63.5189) (-57.0263, -64.1611) (-57.4218, -65.3131) (-57.5, -65.7815) (-57.5, -66.25) knots -2.658203 -2.658203 -2.658203 -2.658203 -2.338234 -2.338234 -2.039357 -2.039357 -1.727845 -1.727845 -1.432975 -1.432975 -1.127717 -1.127717 -0.861349 -0.861349 -0.602484 -0.602484 -0.363754 -0.363754 -0.139905 -0.139905 0 0 0 0
  line L5 (-11.5, -32.75) -> (0.5, -32.75)
  line L6 (0.5, -32.75) -> (0.5, -12.75)
  line L7 (0.5, -12.75, 0) -> (0.5, -12.75, 5.5)
  line L8 (0.5, -12.75, 5.5) -> (0.5, -2.75, 5.5)
  line L9 (0.5, -2.75, 5.5) -> (0.5, -2.75, 12.5)
  line L10 (0.5, -2.75, 12.5) -> (0.5, -12.75, 12.5)
  line L11 (0.5, -12.75, 12.5) -> (0.5, -12.75, 5.5)
  line L12 (0.5, -32.75, 0) -> (0.5, -32.75, 19)
  line L13 (0.5, -32.75, 19) -> (0.5, -30.75, 19)
  line L14 (0.5, -30.75, 19) -> (0.5, -15.75, 19)
  line L15 (0.5, -15.75, 19) -> (0.5, -15.75, 16)
  line L16 (0.5, -15.75, 16) -> (0.5, -30.75, 16)
  line L17 (0.5, -30.75, 16) -> (0.5, -30.75, 19)
  dimension "d56" = 20
  dimension "d57" = 5.5
  dimension "d58" = 10
  dimension "d59" = 7
  dimension "d62" = 19
  dimension "d63" = 2
  dimension "d64" = 15
  dimension "d65" = 3
  constraint coincident S2.start S2.end
  constraint coincident L3 L5.end
  constraint perpendicular L3 L5
  constraint perpendicular L5 L6
  measures "d56" distance of L5.end L6.end
  measures "d62" distance of L5.end L6.start
extrude "Extrude5" cut sketch "Sketch4" along normal blind 25 contours L8 L9 L10 L11 | L14 L15 L16 L17 in plane through (-0.5, 0, 2) normal (-1, 0, 0)
sketch "Sketch5" plane through (0, 0, 2) normal (0, 0, 1) x (-1, 0, 0)
  spline S0 degree 3 poles (-57.5, -3.75) (-57.5, -4.8214) (-57.0766, -5.8872) (-55.6545, -7.3945) (-54.7032, -7.8673) (-52.6712, -8.0877) (-51.5959, -7.8015) (-49.9532, -6.6081) (-49.3675, -5.7408) (-48.879, -3.7915) (-49.0041, -2.711) (-49.8812, -1.0097) (-50.5464, -0.3517) (-51.9328, 0.3441) (-52.5917, 0.5001) (-53.2508, 0.5) knots -2.658203 -2.658203 -2.658203 -2.658203 -2.338234 -2.338234 -2.039357 -2.039357 -1.727845 -1.727845 -1.432975 -1.432975 -1.127717 -1.127717 -0.861349 -0.861349 -0.664467 -0.664467 -0.664467 -0.664467
  spline S1 degree 3 poles (-53.2508, 0.5) (-53.4583, 0.5) (-53.6659, 0.4847) (-54.6621, 0.3375) (-55.4178, -0.008) (-56.5915, -1.0189) (-57.0263, -1.6611) (-57.4218, -2.8131) (-57.5, -3.2815) (-57.5, -3.75) knots -0.664467 -0.664467 -0.664467 -0.664467 -0.602484 -0.602484 -0.363754 -0.363754 -0.139905 -0.139905 0 0 0 0
  line L0 (-53.2508, 0.5) -> (-93, 0.5)
  line L1 (-93, 0.5) -> (-93, -71)
  line L2 (-93, -71) -> (0.5, -71)
  line L3 (0.5, -71) -> (0.5, 0.5)
  line L4 (0.5, 0.5) -> (-53.2508, 0.5)
  spline S2 degree 3 poles (-11.5, -32.75) (-11.5, -33.8214) (-11.0766, -34.8872) (-9.6545, -36.3945) (-8.7032, -36.8673) (-6.6712, -37.0877) (-5.5959, -36.8015) (-3.9532, -35.6081) (-3.3675, -34.7408) (-2.879, -32.7915) (-3.0041, -31.711) (-3.8812, -30.0097) (-4.5464, -29.3517) (-6.1183, -28.5627) (-7.0138, -28.4189) (-8.6621, -28.6625) (-9.4178, -29.008) (-10.5915, -30.0189) (-11.0263, -30.6611) (-11.4218, -31.8131) (-11.5, -32.2815) (-11.5, -32.75) knots -2.658203 -2.658203 -2.658203 -2.658203 -2.338234 -2.338234 -2.039357 -2.039357 -1.727845 -1.727845 -1.432975 -1.432975 -1.127717 -1.127717 -0.861349 -0.861349 -0.602484 -0.602484 -0.363754 -0.363754 -0.139905 -0.139905 0 0 0 0
  spline S3 degree 3 poles (-57.5, -66.25) (-57.5, -67.3214) (-57.0766, -68.3872) (-55.6545, -69.8945) (-54.7032, -70.3673) (-52.6712, -70.5877) (-51.5959, -70.3015) (-49.9532, -69.1081) (-49.3675, -68.2408) (-48.879, -66.2915) (-49.0041, -65.211) (-49.8812, -63.5097) (-50.5464, -62.8517) (-52.1183, -62.0627) (-53.0138, -61.9189) (-54.6621, -62.1625) (-55.4178, -62.508) (-56.5915, -63.5189) (-57.0263, -64.1611) (-57.4218, -65.3131) (-57.5, -65.7815) (-57.5, -66.25) knots -2.658203 -2.658203 -2.658203 -2.658203 -2.338234 -2.338234 -2.039357 -2.039357 -1.727845 -1.727845 -1.432975 -1.432975 -1.127717 -1.127717 -0.861349 -0.861349 -0.602484 -0.602484 -0.363754 -0.363754 -0.139905 -0.139905 0 0 0 0
  line L5 (0.5, -71) -> (-17.5, -71)
  line L6 (-17.5, -71) -> (-17.5, -56)
  line L7 (-17.5, -56) -> (0.5, -56)
  line L8 (0.5, -56) -> (0.5, -71)
  line L9 (-18.5, -56) -> (-76.5, -56)
  line L10 (-76.5, -54) -> (-18.5, -54)
  line L11 (-18.5, -50) -> (-76.5, -50)
  line L12 (-76.5, -48) -> (-18.5, -48)
  line L13 (-18.5, -38) -> (-76.5, -38)
  line L14 (-76.5, -36) -> (-18.5, -36)
  line L15 (-76.5, -42) -> (-18.5, -42)
  line L16 (-18.5, -44) -> (-76.5, -44)
  line L17 (-18.5, -26) -> (-76.5, -26)
  line L18 (-76.5, -30) -> (-18.5, -30)
  line L19 (-76.5, -12) -> (-18.5, -12)
  line L20 (-76.5, -18) -> (-18.5, -18)
  line L21 (-18.5, -14) -> (-76.5, -14)
  line L22 (-76.5, -24) -> (-18.5, -24)
  line L23 (-18.5, -20) -> (-76.5, -20)
  line L24 (-18.5, -32) -> (-76.5, -32)
  arc A0 (-77.5, -55) -> (-76.5, -56) centre (-76.5, -55) ccw
  arc A1 (-76.5, -54) -> (-77.5, -55) centre (-76.5, -55) ccw
  arc A2 (-18.5, -56) -> (-17.5, -55) centre (-18.5, -55) ccw
  arc A3 (-17.5, -55) -> (-18.5, -54) centre (-18.5, -55) ccw
  arc A4 (-18.5, -50) -> (-17.5, -49) centre (-18.5, -49) ccw
  arc A5 (-17.5, -49) -> (-18.5, -48) centre (-18.5, -49) ccw
  arc A6 (-18.5, -44) -> (-17.5, -43) centre (-18.5, -43) ccw
  arc A7 (-17.5, -43) -> (-18.5, -42) centre (-18.5, -43) ccw
  arc A8 (-18.5, -38) -> (-17.5, -37) centre (-18.5, -37) ccw
  arc A9 (-17.5, -37) -> (-18.5, -36) centre (-18.5, -37) ccw
  arc A10 (-18.5, -32) -> (-17.5, -31) centre (-18.5, -31) ccw
  arc A11 (-17.5, -31) -> (-18.5, -30) centre (-18.5, -31) ccw
  arc A12 (-18.5, -26) -> (-17.5, -25) centre (-18.5, -25) ccw
  arc A13 (-17.5, -25) -> (-18.5, -24) centre (-18.5, -25) ccw
  arc A14 (-18.5, -20) -> (-17.5, -19) centre (-18.5, -19) ccw
  arc A15 (-17.5, -19) -> (-18.5, -18) centre (-18.5, -19) ccw
  arc A16 (-18.5, -14) -> (-17.5, -13) centre (-18.5, -13) ccw
  arc A17 (-17.5, -13) -> (-18.5, -12) centre (-18.5, -13) ccw
  arc A18 (-77.5, -49) -> (-76.5, -50) centre (-76.5, -49) ccw
  arc A19 (-76.5, -48) -> (-77.5, -49) centre (-76.5, -49) ccw
  arc A20 (-77.5, -43) -> (-76.5, -44) centre (-76.5, -43) ccw
  arc A21 (-76.5, -42) -> (-77.5, -43) centre (-76.5, -43) ccw
  arc A22 (-77.5, -37) -> (-76.5, -38) centre (-76.5, -37) ccw
  arc A23 (-76.5, -36) -> (-77.5, -37) centre (-76.5, -37) ccw
  arc A24 (-77.5, -31) -> (-76.5, -32) centre (-76.5, -31) ccw
  arc A25 (-76.5, -30) -> (-77.5, -31) centre (-76.5, -31) ccw
  arc A26 (-77.5, -25) -> (-76.5, -26) centre (-76.5, -25) ccw
  arc A27 (-76.5, -24) -> (-77.5, -25) centre (-76.5, -25) ccw
  arc A28 (-77.5, -19) -> (-76.5, -20) centre (-76.5, -19) ccw
  arc A29 (-76.5, -18) -> (-77.5, -19) centre (-76.5, -19) ccw
  arc A30 (-77.5, -13) -> (-76.5, -14) centre (-76.5, -13) ccw
  arc A31 (-76.5, -12) -> (-77.5, -13) centre (-76.5, -13) ccw
  point P0 (-77.5, -56)
  point P1 (-17.5, -54)
  point P2 (-17.5, -48)
  point P3 (-77.5, -50)
  point P4 (-17.5, -50)
  point P5 (-77.5, -38)
  point P6 (-17.5, -36)
  point P7 (-17.5, -38)
  point P8 (-17.5, -42)
  point P9 (-77.5, -44)
  point P10 (-17.5, -44)
  point P11 (-17.5, -18)
  point P12 (-17.5, -20)
  point P13 (-77.5, -20)
  point P14 (-77.5, -26)
  point P15 (-17.5, -24)
  point P16 (-17.5, -26)
  point P17 (-77.5, -14)
  point P18 (-17.5, -12)
  point P19 (-17.5, -14)
  point P20 (-17.5, -30)
  point P21 (-77.5, -32)
  point P22 (-17.5, -32)
  dimension "d66" = 18
  dimension "d67" = 15
  dimension "d68" = 60
  dimension "d69" = 2
  dimension "d70" = 60
  dimension "d71" = 2
  dimension "d72" = 60
  dimension "d73" = 2
  dimension "d74" = 60
  dimension "d75" = 2
  dimension "d76" = 60
  dimension "d77" = 2
  dimension "d78" = 60
  dimension "d79" = 2
  dimension "d80" = 60
  dimension "d81" = 2
  dimension "d82" = 60
  dimension "d83" = 2
  dimension "d84" = 1
  dimension "d85" = 1
  constraint horizontal L5
  constraint vertical L6
  constraint horizontal L7
  constraint vertical L8
  constraint coincident L2.end L3.start
  constraint horizontal L9
  constraint horizontal L10
  constraint horizontal L11
  constraint horizontal L12
  constraint horizontal L16
  constraint horizontal L15
  constraint horizontal L13
  constraint horizontal L14
  constraint horizontal L24
  constraint horizontal L18
  constraint horizontal L17
  constraint horizontal L22
  constraint horizontal L23
  constraint horizontal L20
  constraint horizontal L21
  constraint horizontal L19
  constraint coincident P0 L9
  constraint tangent L9 A0
  constraint tangent L10 A1
  constraint equal A0 A1
  constraint coincident A0.start A1.end
  constraint coincident L6.end L9
  constraint tangent L9 A2
  constraint coincident P1 L10
  constraint tangent L10 A3
  constraint equal A2 A3
  constraint coincident A2.end A3.start
  constraint coincident P4 L11
  constraint tangent L11 A4
  constraint equal A2 A4
  constraint coincident P2 L12
  constraint tangent L12 A5
  constraint equal A2 A5
  constraint coincident A4.end A5.start
  constraint coincident P10 L16
  constraint tangent L16 A6
  constraint equal A2 A6
  constraint coincident P8 L15
  constraint tangent L15 A7
  constraint equal A2 A7
  constraint coincident A6.end A7.start
  constraint coincident P7 L13
  constraint tangent L13 A8
  constraint equal A2 A8
  constraint coincident P6 L14
  constraint tangent L14 A9
  constraint equal A2 A9
  constraint coincident A8.end A9.start
  constraint coincident P22 L24
  constraint tangent L24 A10
  constraint equal A2 A10
  constraint coincident P20 L18
  constraint tangent L18 A11
  constraint equal A2 A11
  constraint coincident A10.end A11.start
  constraint coincident P16 L17
  constraint tangent L17 A12
  constraint equal A2 A12
  constraint coincident P15 L22
  constraint tangent L22 A13
  constraint equal A2 A13
  constraint coincident A12.end A13.start
  constraint coincident P12 L23
  constraint tangent L23 A14
  constraint equal A2 A14
  constraint coincident P11 L20
  constraint tangent L20 A15
  constraint equal A2 A15
  constraint coincident A14.end A15.start
  constraint coincident P19 L21
  constraint tangent L21 A16
  constraint equal A2 A16
  constraint coincident P18 L19
  constraint tangent L19 A17
  constraint equal A2 A17
  constraint coincident A16.end A17.start
  constraint coincident P3 L11
  constraint tangent L11 A18
  constraint equal A2 A18
  constraint tangent L12 A19
  constraint equal A2 A19
  constraint coincident A18.start A19.end
  constraint coincident P9 L16
  constraint tangent L16 A20
  constraint equal A2 A20
  constraint tangent L15 A21
  constraint equal A2 A21
  constraint coincident A20.start A21.end
  constraint coincident P5 L13
  constraint tangent L13 A22
  constraint equal A2 A22
  constraint tangent L14 A23
  constraint equal A2 A23
  constraint coincident A22.start A23.end
  constraint coincident P21 L24
  constraint tangent L24 A24
  constraint equal A2 A24
  constraint tangent L18 A25
  constraint equal A2 A25
  constraint coincident A24.start A25.end
  constraint coincident P14 L17
  constraint tangent L17 A26
  constraint equal A2 A26
  constraint tangent L22 A27
  constraint equal A2 A27
  constraint coincident A26.start A27.end
  constraint coincident P13 L23
  constraint tangent L23 A28
  constraint equal A2 A28
  constraint tangent L20 A29
  constraint equal A2 A29
  constraint coincident A28.start A29.end
  constraint coincident P17 L21
  constraint tangent L21 A30
  constraint equal A2 A30
  constraint tangent L19 A31
  constraint equal A2 A31
  constraint coincident A30.start A31.end
  measures "d66" distance of L6.end L7.end
  measures "d67" distance of L5.end L6.end
  measures "d68" distance of L6.end P0
  measures "d69" distance of L6.end P1
  measures "d70" distance of P3 P4
  measures "d71" distance of P2 P4
  measures "d72" distance of P9 P10
  measures "d73" distance of P8 P10
  measures "d74" distance of P5 P7
  measures "d75" distance of P6 P7
  measures "d76" distance of P21 P22
  measures "d77" distance of P20 P22
  measures "d78" distance of P14 P16
  measures "d79" distance of P15 P16
  measures "d80" distance of P12 P13
  measures "d81" distance of P11 P12
  measures "d82" distance of P17 P19
  measures "d83" distance of P18 P19
  measures "d84" radius of A0
  measures "d85" radius of A2